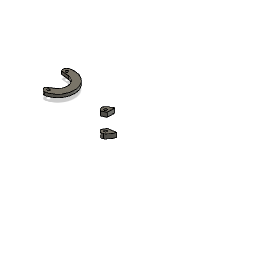
Mounting Locking Bracket - Right (Autodesk Fusion 360 design; units mm, degrees)
Autodesk Fusion 360 part; units mm, degrees
sketch "Sketch1" plane through (-0.1196, 13.2635, 7.5625) normal (0, 1, 0) x (-0.866025, 0, -0.5)
  line L0 (-14.9691, 45.3443) -> (3.1697, 55.8167)
  line L1 (3.1697, 55.8167) -> (3.1697, 146.583)
  arc A0 (3.1697, 146.583) -> (-128.7365, 70.4269) centre (3.6777, -6.6091) ccw
  line L2 (-128.7365, 70.4269) -> (-46.3223, 22.845)
  line L3 (-46.3223, 22.845) -> (-14.9691, 40.9468)
  line L4 (-14.9691, 40.9468) -> (-14.9691, 45.3443)
  line L5 (-8.5758, 68.5574) -> (-16.5936, 66.5924)
  line L6 (-16.5936, 66.5924) -> (-15.0541, 60.3107)
  arc A1 (-15.0541, 60.3107) -> (-44.3999, 43.5674) centre (3.6777, -6.6091) ccw
  line L7 (-44.3999, 43.5674) -> (-48.0269, 48.1063)
  line L8 (-48.0269, 48.1063) -> (-54.4758, 42.9531)
  line L9 (-54.4758, 42.9531) -> (-50.0791, 37.4509)
  arc A2 (-53.7565, 36.9619) -> (-50.0791, 37.4509) centre (-52.2366, 39.6039) ccw
  line L10 (-53.7565, 36.9619) -> (-105.9841, 67.0058)
  spline S0 degree 3 poles (-107.3583, 70.6046) (-107.4828, 70.2277) (-107.5326, 69.8302) (-107.4838, 69.1351) (-107.4188, 68.8413) (-107.3123, 68.5621) (-107.2037, 68.2773) (-107.0516, 68.008) (-106.6228, 67.4609) (-106.323, 67.2008) (-105.9841, 67.0058) knots 0 0 0 0 0.099224 0.099224 0.174187 0.174187 0.174187 0.250654 0.250654 0.348375 0.348375 0.348375 0.348375
  spline S1 degree 3 poles (-107.1901, 71.1894) (-107.1987, 71.1544) (-107.2075, 71.1195) (-107.2467, 70.969) (-107.2717, 70.8666) (-107.3583, 70.6046) knots 0.501684 0.501684 0.501684 0.501684 0.51252 0.51252 0.548438 0.548438 0.548438 0.548438
  line L11 (-107.1901, 71.1894) -> (-102.2708, 72.7276)
  line L12 (-102.2708, 72.7276) -> (-104.6629, 80.378)
  line L13 (-104.6629, 80.378) -> (-109.5822, 78.8398)
  spline S2 degree 3 poles (-110.0536, 79.2247) (-110.0148, 79.1955) (-109.9763, 79.1659) (-109.8164, 79.0408) (-109.6978, 78.942) (-109.5822, 78.8398) knots 0.287713 0.287713 0.287713 0.287713 0.302282 0.302282 0.348613 0.348613 0.348613 0.348613
  spline S3 degree 3 poles (-110.6533, 83.4956) (-110.7036, 83.4289) (-110.751, 83.3604) (-111.0153, 82.9429) (-111.1639, 82.5507) (-111.2777, 81.8453) (-111.281, 81.539) (-111.2388, 81.2372) (-111.2118, 81.0441) (-111.1663, 80.8544) (-111.0025, 80.3769) (-110.856, 80.0975) (-110.4963, 79.6114) (-110.2879, 79.4011) (-110.0536, 79.2247) knots 0 0 0 0 0.020872 0.020872 0.12391 0.12391 0.200135 0.200135 0.200135 0.248905 0.248905 0.326939 0.326939 0.400269 0.400269 0.400269 0.400269
  spline S4 degree 3 poles (-17.2056, 137.5487) (-26.3851, 136.4004) (-35.4111, 134.338) (-52.8908, 128.4648) (-61.3624, 124.643) (-69.3717, 120.0134) (-77.4004, 115.3725) (-84.9462, 109.9359) (-91.8953, 103.7829) (-98.8108, 97.6596) (-105.0939, 90.8631) (-110.6533, 83.4956) knots 0.297101 0.297101 0.297101 0.297101 3.064946 3.064946 5.832791 5.832791 5.832791 8.607361 8.607361 8.607361 11.368481 11.368481 11.368481 11.368481
  spline S5 degree 3 poles (-13.7987, 134.8685) (-13.8553, 135.3661) (-14.036, 135.8464) (-14.4924, 136.5069) (-14.7021, 136.7304) (-14.9416, 136.919) (-15.0928, 137.038) (-15.2545, 137.1422) (-15.6968, 137.3714) (-15.9914, 137.4715) (-16.5944, 137.5786) (-16.9026, 137.5865) (-17.2056, 137.5487) knots 0 0 0 0 0.125191 0.125191 0.201434 0.201434 0.201434 0.249555 0.249555 0.326549 0.326549 0.402867 0.402867 0.402867 0.402867
  spline S6 degree 3 poles (-13.706, 134.2654) (-13.7394, 134.4373) (-13.7719, 134.6322) (-13.7987, 134.8685) knots 0.128256 0.128256 0.128256 0.128256 0.181735 0.181735 0.181735 0.181735
  line L14 (-13.706, 134.2654) -> (-17.5362, 130.7693)
  line L15 (-17.5362, 130.7693) -> (-12.0957, 124.8089)
  line L16 (-12.0957, 124.8089) -> (-8.2656, 128.305)
  spline S7 degree 3 poles (-7.6734, 128.1577) (-7.8577, 128.1959) (-7.948, 128.2191) (-8.124, 128.2649) (-8.1949, 128.2844) (-8.2656, 128.305) knots 0.206215 0.206215 0.206215 0.206215 0.329636 0.329636 0.413668 0.413668 0.413668 0.413668
  spline S8 degree 3 poles (-5.2438, 125.1683) (-5.2432, 125.5652) (-5.3201, 125.9584) (-5.5836, 126.6034) (-5.7371, 126.8623) (-5.9255, 127.0943) (-6.1176, 127.3309) (-6.3462, 127.5391) (-6.9245, 127.925) (-7.2906, 128.0784) (-7.6734, 128.1577) knots 0 0 0 0 0.099224 0.099224 0.174189 0.174189 0.174189 0.250656 0.250656 0.348379 0.348379 0.348379 0.348379
  line L17 (-5.2438, 125.1683) -> (-5.3388, 64.9158)
  arc A3 (-7.0172, 62.1977) -> (-5.3388, 64.9158) centre (-8.3868, 64.9206) ccw
  line L18 (-7.0172, 62.1977) -> (-8.5758, 68.5574)
  circle A4 centre (-114.2687, 72.6834) radius 4.508
  circle A5 centre (-44.0521, 36.0691) radius 4.508
  circle A6 centre (-98.0136, 57.5124) radius 2.413
  circle A7 centre (-72.7366, 42.805) radius 2.413
  circle A8 centre (-52.0375, 31.4587) radius 2.413
  circle A9 centre (-26.3643, 45.4252) radius 8.382
  circle A10 centre (-1.4324, 60.6756) radius 2.413
  circle A11 centre (-0.9091, 84.2747) radius 2.413
  circle A12 centre (-1.0075, 113.5189) radius 2.413
  circle A13 centre (-6.0236, 135.1787) radius 4.508
  circle A14 centre (-9.4154, 56.0666) radius 4.508
  line L19 (-112.0261, 53.2907) -> (-89.8491, 40.4019)
  line L20 (-89.8491, 40.4019) -> (-86.9774, 45.343)
  line L21 (-86.9774, 45.343) -> (-130.0775, 70.3917)
  arc A15 (4.7548, 147.723) -> (-130.0775, 70.3917) centre (3.6777, -6.6091) ccw
  line L22 (4.7548, 147.723) -> (4.612, 97.8964)
  line L23 (4.612, 97.8964) -> (10.3271, 97.8964)
  line L24 (10.3271, 97.8964) -> (10.4002, 123.4298)
  arc A16 (10.4002, 123.4298) -> (10.4258, 132.3532) centre (8.508, 127.8969) ccw
  line L25 (10.4258, 132.3532) -> (10.4857, 153.2969)
  arc A17 (10.4857, 153.2969) -> (-10.2869, 152.8314) centre (3.6777, -6.6091) ccw
  arc A18 (-10.2869, 152.8314) -> (-19.7604, 151.7164) centre (-14.9198, 151.3919) ccw
  arc A19 (-19.7604, 151.7164) -> (-121.1427, 93.5716) centre (3.6777, -6.6091) ccw
  arc A20 (-121.1427, 93.5716) -> (-126.904, 85.9367) centre (-123.3724, 89.263) ccw
  arc A21 (-126.904, 85.9367) -> (-137.7824, 68.2596) centre (3.6777, -6.6091) ccw
  line L26 (-137.7824, 68.2596) -> (-119.7413, 57.7745)
  arc A22 (-119.7413, 57.7745) -> (-112.0261, 53.2907) centre (-114.9265, 57.1796) ccw
  circle A23 centre (-114.9265, 57.1796) radius 2.413
  circle A24 centre (-14.9198, 151.3919) radius 2.413
  circle A25 centre (8.508, 127.8969) radius 2.413
  circle A26 centre (-123.3724, 89.263) radius 2.413
  line L27 (8.508, 127.8969) -> (-14.9198, 151.3919) construction
  circle A27 centre (-3.2059, 139.6444) radius 19.0027
  circle A28 centre (-3.2059, 139.6444) radius 12.1822
  circle A29 centre (-14.9198, 151.3919) radius 1.6
  circle A30 centre (8.508, 127.8969) radius 1.6
  circle A31 centre (-3.2059, 139.6444) radius 21.167
  line L28 (10.4258, 132.3532) -> (1.7219, 128.5034)
  line L29 (-10.2869, 152.8314) -> (-14.1324, 145.0312)
  dimension "d2026" = 3.2
  dimension "d2027" = 3.2
  constraint coincident A16.centre A25.centre
  constraint coincident A18.centre A24.centre
  constraint midpoint L27 A27.centre
  constraint tangent A24 A27
  constraint concentric A27 A28
  constraint concentric A28 A31
  constraint coincident L24.end A31
  constraint coincident A16.end L25.start
  constraint coincident A28 L28.end
  constraint tangent A28 L28
  constraint coincident A17.end A18.start
  constraint coincident A28 L29.end
  constraint tangent A28 L29
  measures "d2026" diameter of A29
  measures "d2027" diameter of A30
extrude "Extrude1" add sketch "Sketch1" along normal blind 3.81 contours L1 L17 A27 A31 | L1 L22 A27 A31 | L1 L14 L15 L16 S7 S8 L17 A27 A28 L28 | L1 L22 A27 L28 | S4 L17 A27 A31 | L22 A16 A27 A31 | S4 S5 L14 L15 L16 S7 S8 L17 A27 A28 | A25 | L22 A16 A27 L28 | A0 S4 A27 A31 | A0 A15 A27 A31 | A0 S4 S5 A27 A28 L29 | A0 A15 A27 L29 | A15 A18 A19 A27 A31 | A24 | A15 A18 A27 L29 | A18 A19 A31 makes body 1
sketch "Sketch2" plane through (0, 13.2635, 0) normal (0, -1, 0) x (1, 0, 0)
  circle A0 centre (14.9198, 151.3919) radius 1.6
  circle A1 centre (-8.508, 127.8969) radius 1.6
  arc A2 (-12.9697, 125.9919) -> (16.812, 155.8591) centre (3.2059, 139.6444) ccw
  arc A3 (16.812, 155.8591) -> (10.2869, 152.8314) centre (14.9198, 151.3919) ccw
  line L0 (10.2869, 152.8314) -> (14.1324, 145.0312)
  arc A4 (-1.7219, 128.5034) -> (14.1324, 145.0312) centre (3.2059, 139.6444) ccw
  line L1 (-1.7219, 128.5034) -> (-10.4258, 132.3532)
  arc A5 (-10.4258, 132.3532) -> (-12.9697, 125.9919) centre (-8.508, 127.8969) ccw
  arc A6 (129.4312, 70.2414) -> (-3.6777, 147.0918) centre (-3.6777, -6.6091) ccw
  arc A7 (129.4312, 70.2414) -> (-3.6777, 147.0918) centre (-3.6777, -6.6091) ccw
  line L2 (-3.6777, 89.9699) -> (-3.6777, 94.7959)
  line L3 (-3.6777, 51.126) -> (-3.6777, 147.0918)
  line L4 (-3.6777, 147.0918) -> (-3.6777, 55.6114)
  line L5 (-3.6777, 55.6114) -> (-3.6777, 51.126)
  arc A8 (128.5652, 69.7414) -> (-3.6777, 146.0918) centre (-3.6777, -6.6091) ccw
  arc A9 (-3.6777, 148.0918) -> (-3.6777, 146.0918) centre (-3.6777, 147.0918) ccw
  arc A10 (23.492, 145.6872) -> (13.0719, 147.1824) centre (-3.6777, -6.6091) ccw
  arc A11 (128.5652, 69.7414) -> (130.2972, 70.7414) centre (129.4312, 70.2414) ccw
  line L6 (-2.6777, 51.126) -> (-2.6777, 147.0918)
  arc A12 (-2.6777, 147.0918) -> (-4.6777, 147.0918) centre (-3.6777, 147.0918) ccw
  line L7 (-4.6777, 129.8108) -> (-4.6777, 120.0003)
  line L8 (-4.6777, 55.6114) -> (-4.6777, 51.126)
  arc A13 (-4.6777, 51.126) -> (-2.6777, 51.126) centre (-3.6777, 51.126) ccw
  constraint concentric A6 A8
  constraint coincident A6.end A7.end
  constraint concentric A7 A10
  constraint coincident A6.start A7.start
  constraint tangent A10 A11
  constraint tangent A9 A10
  constraint tangent A8 A9
  constraint tangent A8 A11
  constraint coincident L0 A10.end
  constraint coincident A2 A10.start
  constraint parallel L3 L6
  constraint parallel L4 L7
  constraint parallel L5 L8
  constraint coincident L3.start L5.end
  constraint tangent L8 A13
  constraint tangent L6 A12
  constraint tangent A12 L7
  constraint tangent L6 A13
  constraint coincident L1 L7.start
  constraint coincident A2 L7.end
extrude "Extrude2" add sketch "Sketch2" along normal blind 5.5118 contours A2 L1 A5 L7 | A2 A3 L0 A10 bodies 1 makes body 2 at (-5.4739, 13.2635, 125.6713) makes body 3 at (19.0569, 13.2635, 149.3395)
